Autodesk Inventor part; units mm, degrees
(part 3 of 3)
  spline S144 degree 3 poles (-72.7019, 7.3694) (-72.7019, 6.6497) (-73.2534, 6.0982) (-73.9731, 6.0982) knots 0 0 0 0 1 1 1 1
  line L1393 (-72.7019, 7.3694) -> (-72.7019, 6.6497) construction
  line L1394 (-72.7019, 6.6497) -> (-73.2534, 6.0982) construction
  line L1395 (-73.2534, 6.0982) -> (-73.9731, 6.0982) construction
  spline S145 degree 3 poles (-73.9731, 6.0982) (-74.6928, 6.0982) (-75.2429, 6.6497) (-75.2429, 7.3694) knots 0 0 0 0 1 1 1 1
  line L1396 (-73.9731, 6.0982) -> (-74.6928, 6.0982) construction
  line L1397 (-74.6928, 6.0982) -> (-75.2429, 6.6497) construction
  line L1398 (-75.2429, 6.6497) -> (-75.2429, 7.3694) construction
  spline S146 degree 3 poles (-75.2429, 7.3694) (-75.2429, 8.0891) (-74.6928, 8.6406) (-73.9731, 8.6406) knots 0 0 0 0 1 1 1 1
  line L1399 (-75.2429, 7.3694) -> (-75.2429, 8.0891) construction
  line L1400 (-75.2429, 8.0891) -> (-74.6928, 8.6406) construction
  line L1401 (-74.6928, 8.6406) -> (-73.9731, 8.6406) construction
  spline S147 degree 3 poles (-73.9731, 8.6406) (-73.2534, 8.6406) (-72.7019, 8.0891) (-72.7019, 7.3694) knots 0 0 0 0 1 1 1 1
  line L1402 (-73.9731, 8.6406) -> (-73.2534, 8.6406) construction
  line L1403 (-73.2534, 8.6406) -> (-72.7019, 8.0891) construction
  line L1404 (-72.7019, 8.0891) -> (-72.7019, 7.3694) construction
  spline S148 degree 3 poles (-46.3996, 18.0009) (-46.3996, 17.1116) (-47.1193, 16.3905) (-48.0086, 16.3905) knots 0 0 0 0 1 1 1 1
  line L1405 (-46.3996, 18.0009) -> (-46.3996, 17.1116) construction
  line L1406 (-46.3996, 17.1116) -> (-47.1193, 16.3905) construction
  line L1407 (-47.1193, 16.3905) -> (-48.0086, 16.3905) construction
  spline S149 degree 3 poles (-48.0086, 16.3905) (-48.8993, 16.3905) (-49.619, 17.1116) (-49.619, 18.0009) knots 0 0 0 0 1 1 1 1
  line L1408 (-48.0086, 16.3905) -> (-48.8993, 16.3905) construction
  line L1409 (-48.8993, 16.3905) -> (-49.619, 17.1116) construction
  line L1410 (-49.619, 17.1116) -> (-49.619, 18.0009) construction
  spline S150 degree 3 poles (-49.619, 18.0009) (-49.619, 18.8902) (-48.8993, 19.6099) (-48.0086, 19.6099) knots 0 0 0 0 1 1 1 1
  line L1411 (-49.619, 18.0009) -> (-49.619, 18.8902) construction
  line L1412 (-49.619, 18.8902) -> (-48.8993, 19.6099) construction
  line L1413 (-48.8993, 19.6099) -> (-48.0086, 19.6099) construction
  spline S151 degree 3 poles (-48.0086, 19.6099) (-47.1193, 19.6099) (-46.3996, 18.8902) (-46.3996, 18.0009) knots 0 0 0 0 1 1 1 1
  line L1414 (-48.0086, 19.6099) -> (-47.1193, 19.6099) construction
  line L1415 (-47.1193, 19.6099) -> (-46.3996, 18.8902) construction
  line L1416 (-46.3996, 18.8902) -> (-46.3996, 18.0009) construction
  spline S152 degree 3 poles (-50.3814, 50.0209) (-50.3814, 49.1316) (-51.1011, 48.4119) (-51.9904, 48.4119) knots 0 0 0 0 1 1 1 1
  line L1417 (-50.3814, 50.0209) -> (-50.3814, 49.1316) construction
  line L1418 (-50.3814, 49.1316) -> (-51.1011, 48.4119) construction
  line L1419 (-51.1011, 48.4119) -> (-51.9904, 48.4119) construction
  spline S153 degree 3 poles (-51.9904, 48.4119) (-52.8797, 48.4119) (-53.6008, 49.1316) (-53.6008, 50.0209) knots 0 0 0 0 1 1 1 1
  line L1420 (-51.9904, 48.4119) -> (-52.8797, 48.4119) construction
  line L1421 (-52.8797, 48.4119) -> (-53.6008, 49.1316) construction
  line L1422 (-53.6008, 49.1316) -> (-53.6008, 50.0209) construction
  spline S154 degree 3 poles (-53.6008, 50.0209) (-53.6008, 50.9102) (-52.8797, 51.6299) (-51.9904, 51.6299) knots 0 0 0 0 1 1 1 1
  line L1423 (-53.6008, 50.0209) -> (-53.6008, 50.9102) construction
  line L1424 (-53.6008, 50.9102) -> (-52.8797, 51.6299) construction
  line L1425 (-52.8797, 51.6299) -> (-51.9904, 51.6299) construction
  spline S155 degree 3 poles (-51.9904, 51.6299) (-51.1011, 51.6299) (-50.3814, 50.9102) (-50.3814, 50.0209) knots 0 0 0 0 1 1 1 1
  line L1426 (-51.9904, 51.6299) -> (-51.1011, 51.6299) construction
  line L1427 (-51.1011, 51.6299) -> (-50.3814, 50.9102) construction
  line L1428 (-50.3814, 50.9102) -> (-50.3814, 50.0209) construction
  spline S156 degree 3 poles (-7.7299, 44.0068) (-7.7299, 43.2871) (-8.2801, 42.7356) (-8.9998, 42.7356) knots 0 0 0 0 1 1 1 1
  line L1429 (-7.7299, 44.0068) -> (-7.7299, 43.2871) construction
  line L1430 (-7.7299, 43.2871) -> (-8.2801, 42.7356) construction
  line L1431 (-8.2801, 42.7356) -> (-8.9998, 42.7356) construction
  spline S157 degree 3 poles (-8.9998, 42.7356) (-9.7208, 42.7356) (-10.271, 43.2871) (-10.271, 44.0068) knots 0 0 0 0 1 1 1 1
  line L1432 (-8.9998, 42.7356) -> (-9.7208, 42.7356) construction
  line L1433 (-9.7208, 42.7356) -> (-10.271, 43.2871) construction
  line L1434 (-10.271, 43.2871) -> (-10.271, 44.0068) construction
  spline S158 degree 3 poles (-10.271, 44.0068) (-10.271, 44.7265) (-9.7208, 45.2766) (-8.9998, 45.2766) knots 0 0 0 0 1 1 1 1
  line L1435 (-10.271, 44.0068) -> (-10.271, 44.7265) construction
  line L1436 (-10.271, 44.7265) -> (-9.7208, 45.2766) construction
  line L1437 (-9.7208, 45.2766) -> (-8.9998, 45.2766) construction
  spline S159 degree 3 poles (-8.9998, 45.2766) (-8.2801, 45.2766) (-7.7299, 44.7265) (-7.7299, 44.0068) knots 0 0 0 0 1 1 1 1
  line L1438 (-8.9998, 45.2766) -> (-8.2801, 45.2766) construction
  line L1439 (-8.2801, 45.2766) -> (-7.7299, 44.7265) construction
  line L1440 (-7.7299, 44.7265) -> (-7.7299, 44.0068) construction
  spline S160 degree 3 poles (52.626, 50.0209) (52.626, 49.1316) (51.9063, 48.4119) (51.017, 48.4119) knots 0 0 0 0 1 1 1 1
  line L1441 (52.626, 50.0209) -> (52.626, 49.1316) construction
  line L1442 (52.626, 49.1316) -> (51.9063, 48.4119) construction
  line L1443 (51.9063, 48.4119) -> (51.017, 48.4119) construction
  spline S161 degree 3 poles (51.017, 48.4119) (50.1277, 48.4119) (49.408, 49.1316) (49.408, 50.0209) knots 0 0 0 0 1 1 1 1
  line L1444 (51.017, 48.4119) -> (50.1277, 48.4119) construction
  line L1445 (50.1277, 48.4119) -> (49.408, 49.1316) construction
  line L1446 (49.408, 49.1316) -> (49.408, 50.0209) construction
  spline S162 degree 3 poles (49.408, 50.0209) (49.408, 50.9102) (50.1277, 51.6299) (51.017, 51.6299) knots 0 0 0 0 1 1 1 1
  line L1447 (49.408, 50.0209) -> (49.408, 50.9102) construction
  line L1448 (49.408, 50.9102) -> (50.1277, 51.6299) construction
  line L1449 (50.1277, 51.6299) -> (51.017, 51.6299) construction
  spline S163 degree 3 poles (51.017, 51.6299) (51.9063, 51.6299) (52.626, 50.9102) (52.626, 50.0209) knots 0 0 0 0 1 1 1 1
  line L1450 (51.017, 51.6299) -> (51.9063, 51.6299) construction
  line L1451 (51.9063, 51.6299) -> (52.626, 50.9102) construction
  line L1452 (52.626, 50.9102) -> (52.626, 50.0209) construction
  spline S164 degree 3 poles (10.271, 44.0068) (10.271, 43.2871) (9.7208, 42.7356) (9.0011, 42.7356) knots 0 0 0 0 1 1 1 1
  line L1453 (10.271, 44.0068) -> (10.271, 43.2871) construction
  line L1454 (10.271, 43.2871) -> (9.7208, 42.7356) construction
  line L1455 (9.7208, 42.7356) -> (9.0011, 42.7356) construction
  spline S165 degree 3 poles (9.0011, 42.7356) (8.28, 42.7356) (7.7299, 43.2871) (7.7299, 44.0068) knots 0 0 0 0 1 1 1 1
  line L1456 (9.0011, 42.7356) -> (8.28, 42.7356) construction
  line L1457 (8.28, 42.7356) -> (7.7299, 43.2871) construction
  line L1458 (7.7299, 43.2871) -> (7.7299, 44.0068) construction
  spline S166 degree 3 poles (7.7299, 44.0068) (7.7299, 44.7265) (8.28, 45.2766) (9.0011, 45.2766) knots 0 0 0 0 1 1 1 1
  line L1459 (7.7299, 44.0068) -> (7.7299, 44.7265) construction
  line L1460 (7.7299, 44.7265) -> (8.28, 45.2766) construction
  line L1461 (8.28, 45.2766) -> (9.0011, 45.2766) construction
  spline S167 degree 3 poles (9.0011, 45.2766) (9.7208, 45.2766) (10.271, 44.7265) (10.271, 44.0068) knots 0 0 0 0 1 1 1 1
  line L1462 (9.0011, 45.2766) -> (9.7208, 45.2766) construction
  line L1463 (9.7208, 45.2766) -> (10.271, 44.7265) construction
  line L1464 (10.271, 44.7265) -> (10.271, 44.0068) construction
  spline S168 degree 3 poles (20.606, 18.0009) (20.606, 17.1116) (19.8863, 16.3905) (18.997, 16.3905) knots 0 0 0 0 1 1 1 1
  line L1465 (20.606, 18.0009) -> (20.606, 17.1116) construction
  line L1466 (20.606, 17.1116) -> (19.8863, 16.3905) construction
  line L1467 (19.8863, 16.3905) -> (18.997, 16.3905) construction
  spline S169 degree 3 poles (18.997, 16.3905) (18.1064, 16.3905) (17.3867, 17.1116) (17.3867, 18.0009) knots 0 0 0 0 1 1 1 1
  line L1468 (18.997, 16.3905) -> (18.1064, 16.3905) construction
  line L1469 (18.1064, 16.3905) -> (17.3867, 17.1116) construction
  line L1470 (17.3867, 17.1116) -> (17.3867, 18.0009) construction
  spline S170 degree 3 poles (17.3867, 18.0009) (17.3867, 18.8902) (18.1064, 19.6099) (18.997, 19.6099) knots 0 0 0 0 1 1 1 1
  line L1471 (17.3867, 18.0009) -> (17.3867, 18.8902) construction
  line L1472 (17.3867, 18.8902) -> (18.1064, 19.6099) construction
  line L1473 (18.1064, 19.6099) -> (18.997, 19.6099) construction
  spline S171 degree 3 poles (18.997, 19.6099) (19.8863, 19.6099) (20.606, 18.8902) (20.606, 18.0009) knots 0 0 0 0 1 1 1 1
  line L1474 (18.997, 19.6099) -> (19.8863, 19.6099) construction
  line L1475 (19.8863, 19.6099) -> (20.606, 18.8902) construction
  line L1476 (20.606, 18.8902) -> (20.606, 18.0009) construction
  spline S172 degree 3 poles (20.606, -18.0009) (20.606, -18.8902) (19.8863, -19.6113) (18.997, -19.6113) knots 0 0 0 0 1 1 1 1
  line L1477 (20.606, -18.0009) -> (20.606, -18.8902) construction
  line L1478 (20.606, -18.8902) -> (19.8863, -19.6113) construction
  line L1479 (19.8863, -19.6113) -> (18.997, -19.6113) construction
  spline S173 degree 3 poles (18.997, -19.6113) (18.1064, -19.6113) (17.3867, -18.8902) (17.3867, -18.0009) knots 0 0 0 0 1 1 1 1
  line L1480 (18.997, -19.6113) -> (18.1064, -19.6113) construction
  line L1481 (18.1064, -19.6113) -> (17.3867, -18.8902) construction
  line L1482 (17.3867, -18.8902) -> (17.3867, -18.0009) construction
  spline S174 degree 3 poles (17.3867, -18.0009) (17.3867, -17.1116) (18.1064, -16.3919) (18.997, -16.3919) knots 0 0 0 0 1 1 1 1
  line L1483 (17.3867, -18.0009) -> (17.3867, -17.1116) construction
  line L1484 (17.3867, -17.1116) -> (18.1064, -16.3919) construction
  line L1485 (18.1064, -16.3919) -> (18.997, -16.3919) construction
  spline S175 degree 3 poles (18.997, -16.3919) (19.8863, -16.3919) (20.606, -17.1116) (20.606, -18.0009) knots 0 0 0 0 1 1 1 1
  line L1486 (18.997, -16.3919) -> (19.8863, -16.3919) construction
  line L1487 (19.8863, -16.3919) -> (20.606, -17.1116) construction
  line L1488 (20.606, -17.1116) -> (20.606, -18.0009) construction
  spline S176 degree 3 poles (52.626, -49.9795) (52.626, -50.8688) (51.9063, -51.5885) (51.017, -51.5885) knots 0 0 0 0 1 1 1 1
  line L1489 (52.626, -49.9795) -> (52.626, -50.8688) construction
  line L1490 (52.626, -50.8688) -> (51.9063, -51.5885) construction
  line L1491 (51.9063, -51.5885) -> (51.017, -51.5885) construction
  spline S177 degree 3 poles (51.017, -51.5885) (50.1277, -51.5885) (49.408, -50.8688) (49.408, -49.9795) knots 0 0 0 0 1 1 1 1
  line L1492 (51.017, -51.5885) -> (50.1277, -51.5885) construction
  line L1493 (50.1277, -51.5885) -> (49.408, -50.8688) construction
  line L1494 (49.408, -50.8688) -> (49.408, -49.9795) construction
  spline S178 degree 3 poles (49.408, -49.9795) (49.408, -49.0902) (50.1277, -48.3705) (51.017, -48.3705) knots 0 0 0 0 1 1 1 1
  line L1495 (49.408, -49.9795) -> (49.408, -49.0902) construction
  line L1496 (49.408, -49.0902) -> (50.1277, -48.3705) construction
  line L1497 (50.1277, -48.3705) -> (51.017, -48.3705) construction
  spline S179 degree 3 poles (51.017, -48.3705) (51.9063, -48.3705) (52.626, -49.0902) (52.626, -49.9795) knots 0 0 0 0 1 1 1 1
  line L1498 (51.017, -48.3705) -> (51.9063, -48.3705) construction
  line L1499 (51.9063, -48.3705) -> (52.626, -49.0902) construction
  line L1500 (52.626, -49.0902) -> (52.626, -49.9795) construction
  spline S180 degree 3 poles (68.2982, 7.3694) (68.2982, 6.6497) (67.7467, 6.0982) (67.027, 6.0982) knots 0 0 0 0 1 1 1 1
  line L1501 (68.2982, 7.3694) -> (68.2982, 6.6497) construction
  line L1502 (68.2982, 6.6497) -> (67.7467, 6.0982) construction
  line L1503 (67.7467, 6.0982) -> (67.027, 6.0982) construction
  spline S181 degree 3 poles (67.027, 6.0982) (66.3073, 6.0982) (65.7558, 6.6497) (65.7558, 7.3694) knots 0 0 0 0 1 1 1 1
  line L1504 (67.027, 6.0982) -> (66.3073, 6.0982) construction
  line L1505 (66.3073, 6.0982) -> (65.7558, 6.6497) construction
  line L1506 (65.7558, 6.6497) -> (65.7558, 7.3694) construction
  spline S182 degree 3 poles (65.7558, 7.3694) (65.7558, 8.0891) (66.3073, 8.6406) (67.027, 8.6406) knots 0 0 0 0 1 1 1 1
  line L1507 (65.7558, 7.3694) -> (65.7558, 8.0891) construction
  line L1508 (65.7558, 8.0891) -> (66.3073, 8.6406) construction
  line L1509 (66.3073, 8.6406) -> (67.027, 8.6406) construction
  spline S183 degree 3 poles (67.027, 8.6406) (67.7467, 8.6406) (68.2982, 8.0891) (68.2982, 7.3694) knots 0 0 0 0 1 1 1 1
  line L1510 (67.027, 8.6406) -> (67.7467, 8.6406) construction
  line L1511 (67.7467, 8.6406) -> (68.2982, 8.0891) construction
  line L1512 (68.2982, 8.0891) -> (68.2982, 7.3694) construction
  spline S184 degree 3 poles (68.2982, -7.3708) (68.2982, -8.0905) (67.7467, -8.6406) (67.027, -8.6406) knots 0 0 0 0 1 1 1 1
  line L1513 (68.2982, -7.3708) -> (68.2982, -8.0905) construction
  line L1514 (68.2982, -8.0905) -> (67.7467, -8.6406) construction
  line L1515 (67.7467, -8.6406) -> (67.027, -8.6406) construction
  spline S185 degree 3 poles (67.027, -8.6406) (66.3073, -8.6406) (65.7558, -8.0905) (65.7558, -7.3708) knots 0 0 0 0 1 1 1 1
  line L1516 (67.027, -8.6406) -> (66.3073, -8.6406) construction
  line L1517 (66.3073, -8.6406) -> (65.7558, -8.0905) construction
  line L1518 (65.7558, -8.0905) -> (65.7558, -7.3708) construction
  spline S186 degree 3 poles (65.7558, -7.3708) (65.7558, -6.6497) (66.3073, -6.0996) (67.027, -6.0996) knots 0 0 0 0 1 1 1 1
  line L1519 (65.7558, -7.3708) -> (65.7558, -6.6497) construction
  line L1520 (65.7558, -6.6497) -> (66.3073, -6.0996) construction
  line L1521 (66.3073, -6.0996) -> (67.027, -6.0996) construction
  spline S187 degree 3 poles (67.027, -6.0996) (67.7467, -6.0996) (68.2982, -6.6497) (68.2982, -7.3708) knots 0 0 0 0 1 1 1 1
  line L1522 (67.027, -6.0996) -> (67.7467, -6.0996) construction
  line L1523 (67.7467, -6.0996) -> (68.2982, -6.6497) construction
  line L1524 (68.2982, -6.6497) -> (68.2982, -7.3708) construction
  spline S188 degree 3 poles (-25.3917, 18.0009) (-25.3917, 17.1116) (-26.1114, 16.3905) (-27.0006, 16.3905) knots 0 0 0 0 1 1 1 1
  line L1525 (-25.3917, 18.0009) -> (-25.3917, 17.1116) construction
  line L1526 (-25.3917, 17.1116) -> (-26.1114, 16.3905) construction
  line L1527 (-26.1114, 16.3905) -> (-27.0006, 16.3905) construction
  spline S189 degree 3 poles (-27.0006, 16.3905) (-27.8899, 16.3905) (-28.611, 17.1116) (-28.611, 18.0009) knots 0 0 0 0 1 1 1 1
  line L1528 (-27.0006, 16.3905) -> (-27.8899, 16.3905) construction
  line L1529 (-27.8899, 16.3905) -> (-28.611, 17.1116) construction
  line L1530 (-28.611, 17.1116) -> (-28.611, 18.0009) construction
  spline S190 degree 3 poles (-28.611, 18.0009) (-28.611, 18.8902) (-27.8899, 19.6099) (-27.0006, 19.6099) knots 0 0 0 0 1 1 1 1
  line L1531 (-28.611, 18.0009) -> (-28.611, 18.8902) construction
  line L1532 (-28.611, 18.8902) -> (-27.8899, 19.6099) construction
  line L1533 (-27.8899, 19.6099) -> (-27.0006, 19.6099) construction
  spline S191 degree 3 poles (-27.0006, 19.6099) (-26.1114, 19.6099) (-25.3917, 18.8902) (-25.3917, 18.0009) knots 0 0 0 0 1 1 1 1
  line L1534 (-27.0006, 19.6099) -> (-26.1114, 19.6099) construction
  line L1535 (-26.1114, 19.6099) -> (-25.3917, 18.8902) construction
  line L1536 (-25.3917, 18.8902) -> (-25.3917, 18.0009) construction
  spline S192 degree 3 poles (-25.3917, -18.0009) (-25.3917, -18.8902) (-26.1114, -19.6113) (-27.0006, -19.6113) knots 0 0 0 0 1 1 1 1
  line L1537 (-25.3917, -18.0009) -> (-25.3917, -18.8902) construction
  line L1538 (-25.3917, -18.8902) -> (-26.1114, -19.6113) construction
  line L1539 (-26.1114, -19.6113) -> (-27.0006, -19.6113) construction
  spline S193 degree 3 poles (-27.0006, -19.6113) (-27.8899, -19.6113) (-28.611, -18.8902) (-28.611, -18.0009) knots 0 0 0 0 1 1 1 1
  line L1540 (-27.0006, -19.6113) -> (-27.8899, -19.6113) construction
  line L1541 (-27.8899, -19.6113) -> (-28.611, -18.8902) construction
  line L1542 (-28.611, -18.8902) -> (-28.611, -18.0009) construction
  spline S194 degree 3 poles (-28.611, -18.0009) (-28.611, -17.1116) (-27.8899, -16.3919) (-27.0006, -16.3919) knots 0 0 0 0 1 1 1 1
  line L1543 (-28.611, -18.0009) -> (-28.611, -17.1116) construction
  line L1544 (-28.611, -17.1116) -> (-27.8899, -16.3919) construction
  line L1545 (-27.8899, -16.3919) -> (-27.0006, -16.3919) construction
  spline S195 degree 3 poles (-27.0006, -16.3919) (-26.1114, -16.3919) (-25.3917, -17.1116) (-25.3917, -18.0009) knots 0 0 0 0 1 1 1 1
  line L1546 (-27.0006, -16.3919) -> (-26.1114, -16.3919) construction
  line L1547 (-26.1114, -16.3919) -> (-25.3917, -17.1116) construction
  line L1548 (-25.3917, -17.1116) -> (-25.3917, -18.0009) construction
  line L1549 (-33.9895, 68.0217) -> (-25.0111, 68.0217)
  line L1550 (-25.0111, 50.0209) -> (-6.5015, 50.0209)
  line L1551 (6.5015, 50.0209) -> (25.0111, 50.0209)
  line L1552 (-6.5015, 50.0209) -> (-6.5015, 60.0168)
  line L1553 (-6.5015, 60.0168) -> (6.5015, 60.0168)
  line L1554 (6.5015, 60.0168) -> (6.5015, 50.0209)
  line L1555 (-25.0111, -67.9804) -> (-33.9895, -67.9804)
  line L1556 (-6.5015, -59.9754) -> (6.5015, -59.9754)
  line L1557 (6.5015, -59.9754) -> (6.5015, -49.9795)
  line L1558 (6.5015, -49.9795) -> (25.0111, -49.9795)
  line L1559 (-25.0111, -49.9795) -> (-6.5015, -49.9795)
  line L1560 (-6.5015, -49.9795) -> (-6.5015, -59.9754)
  line L1561 (-33.9895, 68.0217) -> (-36.9965, 66.4541)
  line L1562 (-36.9965, 66.4541) -> (-39.9195, 64.7183)
  line L1563 (-39.9195, 64.7183) -> (-42.7569, 62.897)
  line L1564 (-42.7569, 62.897) -> (-45.5103, 60.9488)
  line L1565 (-45.5103, 60.9488) -> (-48.1782, 58.8738)
  line L1566 (-48.1782, 58.8738) -> (-50.7206, 56.6705)
  line L1567 (-50.7206, 56.6705) -> (-53.2189, 54.3405)
  line L1568 (-53.2189, 54.3405) -> (-55.5903, 51.9263)
  line L1569 (-55.5903, 51.9263) -> (-57.8363, 49.428)
  line L1570 (-57.8363, 49.428) -> (-59.954, 46.8015)
  line L1571 (-59.954, 46.8015) -> (-61.9863, 44.0909)
  line L1572 (-61.9863, 44.0909) -> (-63.8917, 41.2962)
  line L1573 (-63.8917, 41.2962) -> (-65.6289, 38.3732)
  line L1574 (-65.6289, 38.3732) -> (-67.2807, 35.4503)
  line L1575 (-67.2807, 35.4503) -> (-68.7628, 32.4019)
  line L1576 (-68.7628, 32.4019) -> (-70.1609, 29.3094)
  line L1577 (-70.1609, 29.3094) -> (-71.3893, 26.1755)
  line L1578 (-71.3893, 26.1755) -> (-72.4482, 22.9561)
  line L1579 (-72.4482, 22.9561) -> (-73.3802, 19.6954)
  line L1580 (-73.3802, 19.6954) -> (-74.9892, 18.5083)
  line L1581 (-74.9892, 18.5083) -> (-76.4714, 17.153)
  line L1582 (-76.4714, 17.153) -> (-77.8267, 15.6708)
  line L1583 (-77.8267, 15.6708) -> (-79.0979, 14.1032)
  line L1584 (-79.0979, 14.1032) -> (-80.1995, 12.4101)
  line L1585 (-80.1995, 12.4101) -> (-81.1729, 10.6729)
  line L1586 (-81.1729, 10.6729) -> (-81.9781, 8.8515)
  line L1587 (-81.9781, 8.8515) -> (-82.6137, 6.9461)
  line L1588 (-82.6137, 6.9461) -> (-83.1211, 4.9979)
  line L1589 (-83.1211, 4.9979) -> (-83.4603, 3.007)
  line L1590 (-83.4603, 3.007) -> (-83.6298, 1.0161)
  line L1591 (-83.6298, 1.0161) -> (-83.6298, -0.9748)
  line L1592 (-83.6298, -0.9748) -> (-83.4603, -3.007)
  line L1593 (-83.4603, -3.007) -> (-83.1211, -4.9566)
  line L1594 (-83.1211, -4.9566) -> (-82.6137, -6.9048)
  line L1595 (-82.6137, -6.9048) -> (-81.9781, -8.8102)
  line L1596 (-81.9781, -8.8102) -> (-81.1729, -10.6315)
  line L1597 (-81.1729, -10.6315) -> (-80.1995, -12.4101)
  line L1598 (-80.1995, -12.4101) -> (-79.0979, -14.0618)
  line L1599 (-79.0979, -14.0618) -> (-77.8267, -15.6722)
  line L1600 (-77.8267, -15.6722) -> (-76.4714, -17.1116)
  line L1601 (-76.4714, -17.1116) -> (-74.9892, -18.4669)
  line L1602 (-74.9892, -18.4669) -> (-73.3802, -19.6954)
  line L1603 (-73.3802, -19.6954) -> (-72.4482, -22.9147)
  line L1604 (-72.4482, -22.9147) -> (-71.3466, -26.1341)
  line L1605 (-71.3466, -26.1341) -> (-70.1181, -29.268)
  line L1606 (-70.1181, -29.268) -> (-68.7628, -32.3591)
  line L1607 (-68.7628, -32.3591) -> (-67.2379, -35.4089)
  line L1608 (-67.2379, -35.4089) -> (-65.5862, -38.3319)
  line L1609 (-65.5862, -38.3319) -> (-63.8504, -41.2121)
  line L1610 (-63.8504, -41.2121) -> (-61.9436, -44.0068)
  line L1611 (-61.9436, -44.0068) -> (-59.9113, -46.7174)
  line L1612 (-59.9113, -46.7174) -> (-57.7935, -49.3439)
  line L1613 (-57.7935, -49.3439) -> (-55.5489, -51.8849)
  line L1614 (-55.5489, -51.8849) -> (-53.1761, -54.2991)
  line L1615 (-53.1761, -54.2991) -> (-50.7206, -56.5864)
  line L1616 (-50.7206, -56.5864) -> (-48.1368, -58.7897)
  line L1617 (-48.1368, -58.7897) -> (-45.4676, -60.9074)
  line L1618 (-45.4676, -60.9074) -> (-42.7142, -62.8556)
  line L1619 (-42.7142, -62.8556) -> (-39.8767, -64.6769)
  line L1620 (-39.8767, -64.6769) -> (-36.9965, -66.4128)
  line L1621 (-36.9965, -66.4128) -> (-33.9895, -67.9804)
  line L1622 (34.0322, -67.9804) -> (37.1248, -66.3287)
  line L1623 (37.1248, -66.3287) -> (40.1318, -64.5501)
  line L1624 (40.1318, -64.5501) -> (43.0547, -62.6433)
  line L1625 (43.0547, -62.6433) -> (45.9336, -60.611)
  line L1626 (45.9336, -60.611) -> (48.6456, -58.4078)
  line L1627 (48.6456, -58.4078) -> (51.3134, -56.1204)
  line L1628 (51.3134, -56.1204) -> (53.8545, -53.6649)
  line L1629 (53.8545, -53.6649) -> (56.2686, -51.1225)
  line L1630 (56.2686, -51.1225) -> (58.556, -48.4974)
  line L1631 (58.556, -48.4974) -> (60.7165, -45.744)
  line L1632 (60.7165, -45.744) -> (62.7915, -42.9065)
  line L1633 (62.7915, -42.9065) -> (64.6969, -39.9409)
  line L1634 (64.6969, -39.9409) -> (66.4769, -36.9338)
  line L1635 (66.4769, -36.9338) -> (68.0859, -33.8427)
  line L1636 (68.0859, -33.8427) -> (69.568, -30.666)
  line L1637 (69.568, -30.666) -> (70.9233, -27.4039)
  line L1638 (70.9233, -27.4039) -> (72.109, -24.1005)
  line L1639 (72.109, -24.1005) -> (73.1679, -20.7542)
  line L1640 (73.1679, -20.7542) -> (74.0158, -17.3653)
  line L1641 (74.0158, -17.3653) -> (74.7355, -13.935)
  line L1642 (74.7355, -13.935) -> (75.3284, -10.4619)
  line L1643 (75.3284, -10.4619) -> (75.7103, -6.9889)
  line L1644 (75.7103, -6.9889) -> (75.964, -3.5158)
  line L1645 (75.964, -3.5158) -> (76.0481, 0)
  line L1646 (76.0481, 0) -> (75.964, 3.5144)
  line L1647 (75.964, 3.5144) -> (75.7103, 7.0302)
  line L1648 (75.7103, 7.0302) -> (75.3284, 10.5033)
  line L1649 (75.3284, 10.5033) -> (74.7355, 13.9763)
  line L1650 (74.7355, 13.9763) -> (74.0158, 17.408)
  line L1651 (74.0158, 17.408) -> (73.1679, 20.7956)
  line L1652 (73.1679, 20.7956) -> (72.109, 24.1418)
  line L1653 (72.109, 24.1418) -> (70.9233, 27.4453)
  line L1654 (70.9233, 27.4453) -> (69.568, 30.6647)
  line L1655 (69.568, 30.6647) -> (68.0859, 33.8413)
  line L1656 (68.0859, 33.8413) -> (66.4769, 36.9338)
  line L1657 (66.4769, 36.9338) -> (64.6969, 39.9822)
  line L1658 (64.6969, 39.9822) -> (62.7915, 42.9052)
  line L1659 (62.7915, 42.9052) -> (60.7165, 45.7854)
  line L1660 (60.7165, 45.7854) -> (58.556, 48.496)
  line L1661 (58.556, 48.496) -> (56.2686, 51.1638)
  line L1662 (56.2686, 51.1638) -> (53.8545, 53.7062)
  line L1663 (53.8545, 53.7062) -> (51.3134, 56.1204)
  line L1664 (51.3134, 56.1204) -> (48.6456, 58.4491)
  line L1665 (48.6456, 58.4491) -> (45.9336, 60.6096)
  line L1666 (45.9336, 60.6096) -> (43.0547, 62.6846)
  line L1667 (43.0547, 62.6846) -> (40.1318, 64.5914)
  line L1668 (40.1318, 64.5914) -> (37.1248, 66.37)
  line L1669 (37.1248, 66.37) -> (34.0322, 68.0217)
  line L1670 (-25.0111, 50.0209) -> (-25.0111, 68.0217)
  line L1671 (25.0111, 50.0209) -> (25.0111, 68.0217)
  line L1672 (25.0111, 68.0217) -> (34.0322, 68.0217)
  line L1673 (-25.0111, -67.9804) -> (-25.0111, -49.9795)
  line L1674 (25.0111, -49.9795) -> (25.0111, -67.9804)
  line L1675 (25.0111, -67.9804) -> (34.0322, -67.9804)
  line L1676 (76.0481, 0) -> (-83.6298, 0)
  line L1677 (0, -67.9804) -> (0, 68.0217)
  line L1678 (0, -49.9795) -> (-13.4, -49.9795)
  line L1679 (-13.4, -49.9795) -> (-13.4, -41.3795)
  line L1680 (-13.4, -41.3795) -> (0, -41.3795)
  line L1681 (0, -49.9795) -> (0, -32.5795)
  line L1682 (0, -32.5795) -> (-7.6, -32.5795)
  line L1683 (-7.6, -32.5795) -> (-7.6, -41.3795)
  line L1684 (-7.6, -32.5795) -> (-7.1, -32.5795)
  line L1685 (-7.1, -32.5795) -> (-7.1, -31.5795)
  line L1686 (-7.6, -41.3795) -> (-12.6, -41.3795)
  line L1687 (-12.6, -41.3795) -> (-12.6, -36.3795)
  line L1688 (-12.6, -36.3795) -> (-7.6, -36.3795)
  line L1689 (-7.6, -36.3795) -> (-7.6, -41.3795)
  line L1690 (-13.4, -49.9795) -> (-12.9, -49.9795)
  line L1691 (-12.9, -49.9795) -> (-16.9, -49.9795)
  line L1692 (-13.4, -49.9795) -> (-13.4, -47.9795)
  line L1693 (-13.4, -47.9795) -> (-17.4, -47.9795)
  line L1694 (-17.4, -47.9795) -> (-17.4, -43.9795)
  line L1695 (-17.4, -43.9795) -> (-13.4, -43.9795)
  line L1696 (-13.4, -43.9795) -> (-13.4, -47.9795)
  line L1697 (-16.9, -49.9795) -> (-7.6, -49.9795)
  line L1698 (-7.6, -49.9795) -> (-7.6, -51.9795)
  line L1699 (-7.6, -51.9795) -> (-16.9, -51.9795)
  line L1700 (-16.9, -51.9795) -> (-16.9, -49.9795)
  point P0 (0, 0)
  point P1 (0, 0)
  point P2 (0, 0)
  point P3 (51.017, 50.0209)
  point P4 (51.017, -49.9795)
  point P5 (18.997, -18.0009)
  point P6 (18.997, 18.0009)
  point P7 (9.0011, 44.0068)
  point P8 (10.271, -44.0068)
  point P9 (9.0011, -44.0068)
  point P10 (-8.9998, 44.0068)
  point P11 (67.027, 7.3694)
  point P12 (67.027, -7.3708)
  point P13 (-8.9998, -44.0068)
  dimension "d2" = 13.4
  dimension "d3" = 8.6
  dimension "d4" = 17.4
  dimension "d5" = 7.6
  dimension "d6" = 0.5
  dimension "d7" = 1
  dimension "d10" = 5
  dimension "d11" = 5
  dimension "d12" = 0.5
  dimension "d15" = 2
  dimension "d16" = 4
  dimension "d17" = 4
  constraints: 2226 end point, 20 coincident, 12 point on line, 7 perpendicular, 6 parallel, 5 horizontal, 1 vertical, 588 other
  measures "d2" distance of L1678.start L1678.end
  measures "d3" distance of L1678.end L1679.end
  measures "d4" distance of L1678.start L1681.end
  measures "d5" distance of L1681.end L1682.end
  measures "d6" distance of L1682.end L1684.end
  measures "d7" distance of L1684.end L1685.end
  measures "d10" distance of L1687.end L1688.end
  measures "d11" distance of L1686.end L1687.end
  measures "d12" distance of L1678.end L1690.end
  measures "d15" distance of L1678.end L1692.end
  measures "d16" distance of L1694.end L1695.end
  measures "d17" distance of L1693.end L1694.end
sketch "Sketch2" plane through (0, 0, 0) normal (0, 1, 0) x (-1, 0, 0)
  line L0 (0, -67.9804) -> (0, 68.0217) projected
  line L1 (-25.0111, -49.9795) -> (-6.5015, -49.9795) projected
  line L2 (-25.0111, -67.9804) -> (-25.0111, -49.9795) projected
  line L3 (-6.5015, -49.9795) -> (-6.5015, -59.9754) projected
  line L4 (-6.5015, -59.9754) -> (6.5015, -59.9754) projected
  line L5 (6.5015, -59.9754) -> (6.5015, -49.9795) projected
  line L6 (-8.9998, -44.0068) -> (0, -44.0068)
  line L7 (0, -44.0068) -> (0, -39.7568)
  line L8 (0, -39.7568) -> (-8.9998, -39.7568)
  line L9 (-8.9998, -39.7568) -> (-8.9998, -44.0068)
  line L10 (-8.9998, -44.0068) -> (0, -44.0068)
  line L11 (0, -44.0068) -> (0, -48.2568)
  line L12 (0, -48.2568) -> (-8.9998, -48.2568)
  line L13 (-8.9998, -48.2568) -> (-8.9998, -44.0068)
  line L14 (0, -39.7568) -> (-9.4, -39.7568)
  line L15 (-13.4, -43.7568) -> (-13.4, -44.2568)
  line L16 (-9.4, -48.2568) -> (0, -48.2568)
  line L17 (0, -48.2568) -> (0, -39.7568)
  line L18 (0, -48.2568) -> (-7.5, -48.2568)
  line L19 (0, -39.7568) -> (-7.5, -39.7568)
  line L20 (-7.5, -39.7568) -> (-7.5, -57.0568)
  line L21 (-7.5, -57.0568) -> (0, -57.0568)
  line L22 (0, -57.0568) -> (0, -39.7568)
  arc A0 (-9.4, -39.7568) -> (-13.4, -43.7568) centre (-9.4, -43.7568) ccw
  arc A1 (-13.4, -44.2568) -> (-9.4, -48.2568) centre (-9.4, -44.2568) ccw
  line L23 (0, -39.7568) -> (-6.1, -39.7568)
  line L24 (0, -34.7568) -> (0, -39.7568)
  line L25 (0, -57.0568) -> (0, -30.8568)
  line L26 (0, -30.8568) -> (-6.1, -30.8568)
  line L27 (-6.1, -30.8568) -> (-6.1, -39.7568)
  line L28 (-6.1, -39.7568) -> (0, -39.7568)
  line L29 (0, -39.7568) -> (0, -30.8568)
  point P0 (0, 0)
  point P1 (-13.4, -48.2568)
  dimension "d18" = 4.25
  dimension "d19" = 4.25
  dimension "d20" = 13.4
  dimension "d23" = 17.3
  dimension "d24" = 7.5
  dimension "d25" = 4
  dimension "d28" = 26.2
  dimension "d29" = 6.1
  constraints: 48 end point, 10 parallel, 7 horizontal, 6 point on line, 5 perpendicular, 4 point on circle, 4 tangent, 2 centre point, 1 equal radius
  measures "d18" distance of L7.end L6.end
  measures "d19" distance of L10.end L11.end
  measures "d20" distance of L16.end point (-13.4, -48.257)
  measures "d23" distance of L20.end L19.end
  measures "d24" distance between parallel lines of L22 L20
  measures "d25" radius of A0
  measures "d28" distance of L21.end L25.end
  measures "d29" distance of L28.end L23.end
sketch "Sketch3" plane through (0, 0, 0) normal (0, 1, 0) x (-1, 0, 0)
  line L0 (0, -67.9804) -> (0, 68.0217) projected
  line L1 (0, -30.8568) -> (-6.1, -30.8568) projected
  line L2 (0, -39.7568) -> (-9.4, -39.7568) projected
  arc A0 (-9.4, -39.7568) -> (-13.4, -43.7568) centre (-9.4, -43.7568) ccw projected
  arc A1 (-13.4, -44.2568) -> (-9.4, -48.2568) centre (-9.4, -44.2568) ccw projected
  line L3 (0, -48.2568) -> (-8.9998, -48.2568) projected
  line L4 (-7.5, -57.0568) -> (0, -57.0568) projected
  line L5 (-6.5015, -49.9795) -> (-6.5015, -59.9754) projected
  line L6 (-6.5015, -59.9754) -> (6.5015, -59.9754) projected
  line L7 (-25.0111, -49.9795) -> (-6.5015, -49.9795) projected
  line L8 (-25.0111, -67.9804) -> (-25.0111, -49.9795) projected
  line L9 (0, -30.8568) -> (-1.5, -30.8568)
  line L10 (-2, -30.3568) -> (-2, -26.3568)
  line L11 (-1.5, -25.8568) -> (0, -25.8568)
  line L12 (0, -25.8568) -> (0, -30.8568)
  arc A2 (-1.5, -25.8568) -> (-2, -26.3568) centre (-1.5, -26.3568) ccw
  arc A3 (-2, -30.3568) -> (-1.5, -30.8568) centre (-1.5, -30.3568) ccw
  line L13 (-6.6, -39.7568) -> (-10.6, -39.7568)
  line L14 (-11.1, -39.2568) -> (-11.1, -31.3568)
  line L15 (-10.6, -30.8568) -> (-6.6, -30.8568)
  arc A4 (-6.1, -31.3568) -> (-6.6, -30.8568) centre (-6.6, -31.3568) ccw
  arc A5 (-10.6, -30.8568) -> (-11.1, -31.3568) centre (-10.6, -31.3568) ccw
  arc A6 (-11.1, -39.2568) -> (-10.6, -39.7568) centre (-10.6, -39.2568) ccw
  arc A7 (-6.6, -39.7568) -> (-6.1, -39.2568) centre (-6.6, -39.2568) ccw
  line L16 (-8.1, -48.2568) -> (-13, -48.2568)
  line L17 (-13.5, -48.2568) -> (-13.5, -51.9795)
  line L18 (-13.5, -51.9795) -> (-8.1, -51.9795)
  line L19 (-7.5, -48.2568) -> (-13.5, -48.2568)
  line L20 (-13.5, -48.7568) -> (-13.5, -48.9795)
  line L21 (-13.5, -49.9795) -> (-7.5, -49.9795)
  line L22 (-17.0198, -49.9795) -> (-24.5111, -49.9795)
  line L23 (-25.0111, -50.4795) -> (-25.0111, -51.4795)
  line L24 (-24.5111, -51.9795) -> (-7.5, -51.9795)
  arc A8 (-7.6, -48.7568) -> (-8.1, -48.2568) centre (-8.1, -48.7568) ccw
  arc A9 (-8.1, -51.9795) -> (-7.6, -51.4795) centre (-8.1, -51.4795) ccw
  arc A10 (-24.5111, -49.9795) -> (-25.0111, -50.4795) centre (-24.5111, -50.4795) ccw
  arc A11 (-25.0111, -51.4795) -> (-24.5111, -51.9795) centre (-24.5111, -51.4795) ccw
  line L25 (-13.5, -48.2568) -> (-16.0198, -49.7116)
  line L26 (-13.5, -48.2568) -> (-10.5904, -48.2568) construction
  arc A12 (-17.0198, -49.9795) -> (-16.0198, -49.7116) centre (-17.0198, -47.9795) ccw
  line L27 (-8.1, -48.2568) -> (-13.5, -48.2568)
  line L28 (-17.0198, -49.9795) -> (-24.5111, -49.9795)
  line L29 (-25.0111, -50.4795) -> (-25.0111, -51.4795)
  line L30 (-24.5111, -51.9795) -> (-8.1, -51.9795)
  line L31 (-6.1, -31.3568) -> (-6.1, -39.2568)
  line L32 (-7.6, -48.7568) -> (-7.6, -51.4795)
  point P0 (0, 0)
  point P1 (-6.1, -39.7568)
  point P2 (-2, -25.8568)
  point P3 (-2, -30.8568)
  point P4 (-11.1, -30.8568)
  point P5 (-6.1, -30.8568)
  point P6 (-7.5, -51.9795)
  point P7 (-25.0111, -51.9795)
  dimension "d30" = 2
  dimension "d31" = 5
  dimension "d32" = 0.5
  dimension "d33" = 5
  dimension "d34" = 0.5
  dimension "d36" = 2
  dimension "d37" = 0.5
  dimension "d40" = 150
  dimension "d41" = 2
  dimension "d47" = 6.1
  dimension "d48" = 7.6
  constraints: 48 end point, 24 tangent, 22 point on circle, 20 point on line, 11 centre point, 6 horizontal, 6 parallel, 6 perpendicular, 5 equal radius, 4 collinear, 1 equal length, 1 vertical
  measures "d30" distance of point (-2, -25.857) L11.end
  measures "d31" distance of point (-2, -30.857) point (-2, -25.857)
  measures "d32" radius of A2
  measures "d33" distance of point (-11.1, -30.857) point (-6.1, -30.857)
  measures "d34" radius of A4
  measures "d36" distance between parallel lines of L7 L18
  measures "d37" radius of A8
  measures "d40" angle of L25 L26
  measures "d41" radius of A12
  measures "d47" distance between parallel lines of L31 L0
  measures "d48" distance between parallel lines of L0 L32
extrude "Extrusion1" add sketch "Sketch3" along normal blind 11.5 contours A8 L32 L7 L17 L19 L16 L3 | L32 A9 L18 L17 L7 | L17 L24 A11 L8 A10 L7 | L7 A12 L25 L17 | L1 A3 L10 A2 L11 L0 | L2 L13 A6 L14 A5 L15 A4 L31 A7
chamfer "Chamfer1" distance 0.5 angle 45 24 edges at (11.1, 11.5, -35.3068) (10.9536, 11.5, -39.6103) (8.6, 11.5, -39.7568) (6.2464, 11.5, -39.6103) (6.1, 11.5, -35.3068) (6.2464, 11.5, -31.0032) (8.6, 11.5, -30.8568) (10.9536, 11.5, -31.0032) (2, 11.5, -28.3568) (1.8536, 11.5, -30.7103) (0.75, 11.5, -30.8568) (1.8536, 11.5, -26.0032) (0.75, 11.5, -25.8568) (14.7599, 11.5, -48.9842) (16.5021, 11.5, -49.9114) (20.7654, 11.5, -49.9795) (24.8647, 11.5, -50.126) (25.0111, 11.5, -50.9795) (24.8647, 11.5, -51.8331) (16.3056, 11.5, -51.9795) (7.7464, 11.5, -51.8331) (7.6, 11.5, -50.1181) (7.7464, 11.5, -48.4032) (10.8, 11.5, -48.2568)
sketch "Sketch5" plane through (0, 0, 0) normal (0, -1, 0) x (1, 0, 0)
  line L0 (0, -30.8568) -> (0, -25.8568) projected
  line L1 (25.0111, -51.9795) -> (0, -51.9795)
  line L2 (0, -51.9795) -> (0, -25.8568)
  line L3 (0, -25.8568) -> (25.0111, -25.8568)
  line L4 (25.0111, -25.8568) -> (25.0111, -51.9795)
  point P0 (0, 0)
  constraints: 8 end point, 2 parallel, 1 horizontal, 1 perpendicular
extrude "Extrusion3" add sketch "Sketch5" along normal blind 2
mirror "Mirror2" about plane through (0, 0, -30.8568) normal (-1, 0, 0) of "Extrusion1", "Chamfer1", "Extrusion3"
body "Solid1"
